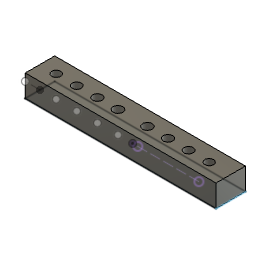
HoleTest v1 (Autodesk Fusion 360 design; units mm, degrees)
Autodesk Fusion 360 part; units mm, degrees
note: some values were not read from the file. Set by a fixed rule: the direction of a hole.
sketch "Sketch1" plane through (0, 0, 0) normal (0, 1, 0) x (1, 0, 0)
  line L0 (-31.5, 5) -> (33.3053, 5)
  line L1 (33.3053, 5) -> (33.3053, -5)
  line L2 (33.3053, -5) -> (-31.5, -5)
  line L3 (-31.5, -5) -> (-31.5, 5)
  line L4 (-31.5, 0) -> (-36.5072, 0) construction
  line L5 (1.75, 0) -> (22.5, 0) construction
  point P0 (-26, 0)
  point P1 (-19, 0)
  point P2 (-12, 0)
  point P3 (-5, 0)
  point P4 (-31.5, 0)
  dimension "d6" = 7
  dimension "d7" = 0
  dimension "d21" = 5
  dimension "d22" = 5.5
  dimension "d23" = 10
  constraint horizontal L0
  constraint perpendicular L0 L1
  constraint parallel L0 L2
  constraint parallel L1 L3
  constraint midpoint L3 P4
  constraint coincident P4 L4.start
  constraint perpendicular L3 L4
  constraint collinear L4 L5
  measures "d21" distance of origin P3
  measures "d22" distance of P0 P4
  measures "d23" distance of L0.end L1.end
extrude "Extrude1" add sketch "Sketch1" along normal blind 7.5
hole "Hole1" at (-26, 0, 0) direction (0, 1, 0) diameter 3 end up to surface (7.5 mm away)
hole "Hole2" at (-19, 0, 0) direction (0, 1, 0) diameter 3.1 end up to surface (7.5 mm away)
hole "Hole3" at (-12, 0, 0) direction (0, 1, 0) diameter 3.2 end up to surface (7.5 mm away)
hole "Hole4" at (-5, 0, 0) direction (0, 1, 0) diameter 3.3 end up to surface (7.5 mm away)
mirror "Mirror1" about plane through (0, 0, 0) normal (1, 0, 0) of "Hole1", "Hole2", "Hole3", "Hole4"
